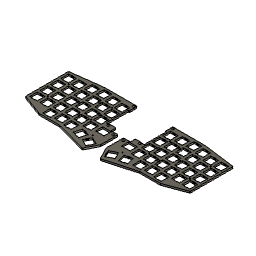
Sofle_Pico_v3.5.5_fdm_notched_plates (Autodesk Fusion 360 design; units mm, degrees)
Autodesk Fusion 360 part; units mm, degrees
sketch "Sketch1" plane through (0, 0, 0) normal (0, 0, 1) x (1, 0, 0)
  line L0 (67.7713, -100.8243) -> (105.871, -100.8243)
  line L1 (0.0502, -63.5467) -> (0.0502, -93.6294)
  arc A0 (12.757, -116.3198) -> (11.0246, -115.5539) centre (12.3611, -114.8731) cw
  arc A1 (28.6597, -14.02) -> (27.6597, -13.02) centre (28.6597, -13.02) cw
  arc A2 (27.6597, -1.075) -> (28.6597, -0.0749) centre (28.6598, -1.075) cw
  line L2 (12.7469, -62.5467) -> (12.7469, -54.5297)
  line L3 (29.4468, -54.1629) -> (29.4468, -14.02)
  line L4 (25.4468, -53.5297) -> (13.7469, -53.5297)
  line L5 (86.8212, -0.075) -> (144.1346, -7.4739)
  line L6 (105.871, -100.8243) -> (144.565, -86.5517)
  line L7 (29.4468, -54.1629) -> (26.3075, -54.1629)
  arc A3 (144.1346, -7.4739) -> (145.4707, -8.9749) centre (143.9598, -8.9748) cw
  line L8 (145.4707, -8.9749) -> (145.4707, -85.1744)
  line L9 (0.2137, -94.3371) -> (11.0246, -115.5539)
  arc A4 (12.7469, -54.5297) -> (13.7469, -53.5297) centre (13.7469, -54.5297) cw
  line L10 (1.0502, -62.5467) -> (12.7469, -62.5467)
  arc A5 (25.4468, -53.5297) -> (26.3075, -54.1629) centre (23.7986, -56.6716) cw
  line L11 (28.6597, -14.02) -> (29.4468, -14.02)
  line L12 (86.8212, -0.075) -> (28.6597, -0.075)
  arc A6 (0.2137, -94.3371) -> (0.0502, -93.6294) centre (1.5521, -93.6552) cw
  line L13 (12.757, -116.3198) -> (67.7713, -100.8243)
  line L14 (27.6597, -1.075) -> (27.6597, -13.02)
  arc A7 (145.4707, -85.1744) -> (144.565, -86.5517) centre (143.9712, -85.1747) cw
  arc A8 (0.0502, -63.5467) -> (1.0502, -62.5468) centre (1.0502, -63.5468) cw
  circle A9 centre (48.7216, -47.4698) radius 1.75
  circle A10 centre (67.7715, -28.4199) radius 1.75
  circle A11 centre (67.7715, -66.5196) radius 1.75
  circle A12 centre (86.8214, -47.4698) radius 1.75
  line L15 (26.6468, -77.0995) -> (11.0469, -77.0995)
  line L16 (11.0469, -77.0995) -> (11.0469, -64.0996)
  line L17 (11.0469, -64.0996) -> (26.6468, -64.0996)
  line L18 (26.6468, -64.0996) -> (26.6468, -77.0995)
  circle A13 centre (124.9361, -28.0099) radius 1.1
  circle A14 centre (124.9211, -66.1246) radius 1.1
  circle A15 centre (48.0866, -25.6099) radius 1.1
  circle A16 centre (48.1766, -63.5596) radius 1.1
  circle A17 centre (22.2368, -86.6295) radius 1.1
  circle A18 centre (30.6568, -3.2176) radius 2.05
  circle A19 centre (23.7868, -56.6897) radius 2.05
  circle A20 centre (4.296, -67.0996) radius 2.05
  line L19 (37.0467, -9.6) -> (41.3467, -9.6)
  line L20 (41.3467, -9.6) -> (41.3467, -8.6)
  line L21 (41.3467, -8.6) -> (37.0467, -8.6)
  line L22 (37.0467, -8.6) -> (37.0467, -9.6)
  line L23 (37.0467, -23.5999) -> (41.3467, -23.5999)
  line L24 (41.3467, -23.5999) -> (41.3467, -22.5999)
  line L25 (41.3467, -22.5999) -> (37.0467, -22.5999)
  line L26 (37.0467, -22.5999) -> (37.0467, -23.5999)
  line L27 (46.1967, -23.0999) -> (32.1968, -23.0999)
  line L28 (32.1968, -23.0999) -> (32.1968, -9.1)
  line L29 (32.1968, -9.1) -> (46.1967, -9.1)
  line L30 (46.1967, -9.1) -> (46.1967, -23.0999)
  line L31 (75.1465, -4.6001) -> (79.4464, -4.6001)
  line L32 (79.4464, -4.6001) -> (79.4464, -3.6001)
  line L33 (79.4464, -3.6001) -> (75.1465, -3.6001)
  line L34 (75.1465, -3.6001) -> (75.1465, -4.6001)
  line L35 (75.1465, -18.6) -> (79.4464, -18.6)
  line L36 (79.4464, -18.6) -> (79.4464, -17.6)
  line L37 (79.4464, -17.6) -> (75.1465, -17.6)
  line L38 (75.1465, -17.6) -> (75.1465, -18.6)
  line L39 (84.2964, -18.1) -> (70.2965, -18.1)
  line L40 (70.2965, -18.1) -> (70.2965, -4.1001)
  line L41 (70.2965, -4.1001) -> (84.2964, -4.1001)
  line L42 (84.2964, -4.1001) -> (84.2964, -18.1)
  line L43 (37.0467, -47.6998) -> (41.3467, -47.6998)
  line L44 (41.3467, -47.6998) -> (41.3467, -46.6998)
  line L45 (41.3467, -46.6998) -> (37.0467, -46.6998)
  line L46 (37.0467, -46.6998) -> (37.0467, -47.6998)
  line L47 (37.0467, -61.6997) -> (41.3467, -61.6997)
  line L48 (41.3467, -61.6997) -> (41.3467, -60.6997)
  line L49 (41.3467, -60.6997) -> (37.0467, -60.6997)
  line L50 (37.0467, -60.6997) -> (37.0467, -61.6997)
  line L51 (46.1967, -61.1997) -> (32.1968, -61.1997)
  line L52 (32.1968, -61.1997) -> (32.1968, -47.1998)
  line L53 (32.1968, -47.1998) -> (46.1967, -47.1998)
  line L54 (46.1967, -47.1998) -> (46.1967, -61.1997)
  line L55 (56.0966, -45.1998) -> (60.3966, -45.1998)
  line L56 (60.3966, -45.1998) -> (60.3966, -44.1998)
  line L57 (60.3966, -44.1998) -> (56.0966, -44.1998)
  line L58 (56.0966, -44.1998) -> (56.0966, -45.1998)
  line L59 (56.0966, -59.1997) -> (60.3966, -59.1997)
  line L60 (60.3966, -59.1997) -> (60.3966, -58.1997)
  line L61 (60.3966, -58.1997) -> (56.0966, -58.1997)
  line L62 (56.0966, -58.1997) -> (56.0966, -59.1997)
  line L63 (65.2465, -58.6997) -> (51.2466, -58.6997)
  line L64 (51.2466, -58.6997) -> (51.2466, -44.6998)
  line L65 (51.2466, -44.6998) -> (65.2465, -44.6998)
  line L66 (65.2465, -44.6998) -> (65.2465, -58.6997)
  line L67 (75.1465, -61.7496) -> (79.4464, -61.7496)
  line L68 (79.4464, -61.7496) -> (79.4464, -60.7497)
  line L69 (79.4464, -60.7497) -> (75.1465, -60.7497)
  line L70 (75.1465, -60.7497) -> (75.1465, -61.7496)
  line L71 (75.1465, -75.7495) -> (79.4464, -75.7495)
  line L72 (79.4464, -75.7495) -> (79.4464, -74.7496)
  line L73 (79.4464, -74.7496) -> (75.1465, -74.7496)
  line L74 (75.1465, -74.7496) -> (75.1465, -75.7495)
  line L75 (84.2964, -75.2496) -> (70.2965, -75.2496)
  line L76 (70.2965, -75.2496) -> (70.2965, -61.2497)
  line L77 (70.2965, -61.2497) -> (84.2964, -61.2497)
  line L78 (84.2964, -61.2497) -> (84.2964, -75.2496)
  line L79 (113.2462, -69.1496) -> (117.5461, -69.1496)
  line L80 (117.5461, -69.1496) -> (117.5461, -68.1496)
  line L81 (117.5461, -68.1496) -> (113.2462, -68.1496)
  line L82 (113.2462, -68.1496) -> (113.2462, -69.1496)
  line L83 (113.2462, -83.1495) -> (117.5461, -83.1495)
  line L84 (117.5461, -83.1495) -> (117.5461, -82.1495)
  line L85 (117.5461, -82.1495) -> (113.2462, -82.1495)
  line L86 (113.2462, -82.1495) -> (113.2462, -83.1495)
  line L87 (122.3961, -82.6495) -> (108.3962, -82.6495)
  line L88 (108.3962, -82.6495) -> (108.3962, -68.6496)
  line L89 (108.3962, -68.6496) -> (122.3961, -68.6496)
  line L90 (122.3961, -68.6496) -> (122.3961, -82.6495)
  line L91 (20.2581, -95.0736) -> (22.2101, -98.905)
  line L92 (22.2101, -98.905) -> (23.1011, -98.451)
  line L93 (23.1011, -98.451) -> (21.149, -94.6197)
  line L94 (21.149, -94.6197) -> (20.2581, -95.0736)
  line L95 (7.784, -101.4295) -> (9.7361, -105.2607)
  line L96 (9.7361, -105.2607) -> (10.6271, -104.8067)
  line L97 (10.6271, -104.8067) -> (8.675, -100.9755)
  line L98 (8.675, -100.9755) -> (7.784, -101.4295)
  line L99 (12.3835, -109.3551) -> (6.0277, -96.8811)
  line L100 (6.0277, -96.8811) -> (18.5017, -90.5253)
  line L101 (18.5017, -90.5253) -> (24.8575, -102.9993)
  line L102 (24.8575, -102.9993) -> (12.3835, -109.3551)
  line L103 (32.4877, -88.7775) -> (36.6411, -87.6646)
  line L104 (36.6411, -87.6646) -> (36.3823, -86.6986)
  line L105 (36.3823, -86.6986) -> (32.2289, -87.8116)
  line L106 (32.2289, -87.8116) -> (32.4877, -88.7775)
  line L107 (36.1111, -102.3003) -> (40.2645, -101.1874)
  line L108 (40.2645, -101.1874) -> (40.0057, -100.2215)
  line L109 (40.0057, -100.2215) -> (35.8522, -101.3344)
  line L110 (35.8522, -101.3344) -> (36.1111, -102.3003)
  line L111 (44.8199, -99.4492) -> (31.297, -103.0726)
  line L112 (31.297, -103.0726) -> (27.6735, -89.5497)
  line L113 (27.6735, -89.5497) -> (41.1964, -85.9263)
  line L114 (41.1964, -85.9263) -> (44.8199, -99.4492)
  line L115 (132.296, -31.0499) -> (136.596, -31.0499)
  line L116 (136.596, -31.0499) -> (136.596, -30.0499)
  line L117 (136.596, -30.0499) -> (132.296, -30.0499)
  line L118 (132.296, -30.0499) -> (132.296, -31.0499)
  line L119 (132.296, -45.0498) -> (136.596, -45.0498)
  line L120 (136.596, -45.0498) -> (136.596, -44.0498)
  line L121 (136.596, -44.0498) -> (132.296, -44.0498)
  line L122 (132.296, -44.0498) -> (132.296, -45.0498)
  line L123 (141.446, -44.5498) -> (127.4461, -44.5498)
  line L124 (127.4461, -44.5498) -> (127.4461, -30.5499)
  line L125 (127.4461, -30.5499) -> (141.446, -30.5499)
  line L126 (141.446, -30.5499) -> (141.446, -44.5498)
  line L127 (132.296, -50.0997) -> (136.596, -50.0997)
  line L128 (136.596, -50.0997) -> (136.596, -49.0997)
  line L129 (136.596, -49.0997) -> (132.296, -49.0997)
  line L130 (132.296, -49.0997) -> (132.296, -50.0997)
  line L131 (132.296, -64.0996) -> (136.596, -64.0996)
  line L132 (136.596, -64.0996) -> (136.596, -63.0996)
  line L133 (136.596, -63.0996) -> (132.296, -63.0996)
  line L134 (132.296, -63.0996) -> (132.296, -64.0996)
  line L135 (141.446, -63.5996) -> (127.4461, -63.5996)
  line L136 (127.4461, -63.5996) -> (127.4461, -49.5997)
  line L137 (127.4461, -49.5997) -> (141.446, -49.5997)
  line L138 (141.446, -49.5997) -> (141.446, -63.5996)
  line L139 (132.296, -69.1496) -> (136.596, -69.1496)
  line L140 (136.596, -69.1496) -> (136.596, -68.1496)
  line L141 (136.596, -68.1496) -> (132.296, -68.1496)
  line L142 (132.296, -68.1496) -> (132.296, -69.1496)
  line L143 (132.296, -83.1495) -> (136.596, -83.1495)
  line L144 (136.596, -83.1495) -> (136.596, -82.1495)
  line L145 (136.596, -82.1495) -> (132.296, -82.1495)
  line L146 (132.296, -82.1495) -> (132.296, -83.1495)
  line L147 (141.446, -82.6495) -> (127.4461, -82.6495)
  line L148 (127.4461, -82.6495) -> (127.4461, -68.6496)
  line L149 (127.4461, -68.6496) -> (141.446, -68.6496)
  line L150 (141.446, -68.6496) -> (141.446, -82.6495)
  line L151 (94.1963, -7.1) -> (98.4963, -7.1)
  line L152 (98.4963, -7.1) -> (98.4963, -6.1001)
  line L153 (98.4963, -6.1001) -> (94.1963, -6.1001)
  line L154 (94.1963, -6.1001) -> (94.1963, -7.1)
  line L155 (94.1963, -21.0999) -> (98.4963, -21.0999)
  line L156 (98.4963, -21.0999) -> (98.4963, -20.1)
  line L157 (98.4963, -20.1) -> (94.1963, -20.1)
  line L158 (94.1963, -20.1) -> (94.1963, -21.0999)
  line L159 (103.3462, -20.5999) -> (89.3463, -20.5999)
  line L160 (89.3463, -20.5999) -> (89.3463, -6.6001)
  line L161 (89.3463, -6.6001) -> (103.3462, -6.6001)
  line L162 (103.3462, -6.6001) -> (103.3462, -20.5999)
  line L163 (113.2462, -12) -> (117.5461, -12)
  line L164 (117.5461, -12) -> (117.5461, -11)
  line L165 (117.5461, -11) -> (113.2462, -11)
  line L166 (113.2462, -11) -> (113.2462, -12)
  line L167 (113.2462, -25.9999) -> (117.5461, -25.9999)
  line L168 (117.5461, -25.9999) -> (117.5461, -24.9999)
  line L169 (117.5461, -24.9999) -> (113.2462, -24.9999)
  line L170 (113.2462, -24.9999) -> (113.2462, -25.9999)
  line L171 (122.3961, -25.4999) -> (108.3962, -25.4999)
  line L172 (108.3962, -25.4999) -> (108.3962, -11.5)
  line L173 (108.3962, -11.5) -> (122.3961, -11.5)
  line L174 (122.3961, -11.5) -> (122.3961, -25.4999)
  line L175 (56.0966, -26.1499) -> (60.3966, -26.1499)
  line L176 (60.3966, -26.1499) -> (60.3966, -25.1499)
  line L177 (60.3966, -25.1499) -> (56.0966, -25.1499)
  line L178 (56.0966, -25.1499) -> (56.0966, -26.1499)
  line L179 (56.0966, -40.1498) -> (60.3966, -40.1498)
  line L180 (60.3966, -40.1498) -> (60.3966, -39.1498)
  line L181 (60.3966, -39.1498) -> (56.0966, -39.1498)
  line L182 (56.0966, -39.1498) -> (56.0966, -40.1498)
  line L183 (65.2465, -39.6498) -> (51.2466, -39.6498)
  line L184 (51.2466, -39.6498) -> (51.2466, -25.6499)
  line L185 (51.2466, -25.6499) -> (65.2465, -25.6499)
  line L186 (65.2465, -25.6499) -> (65.2465, -39.6498)
  line L187 (94.1963, -26.1499) -> (98.4963, -26.1499)
  line L188 (98.4963, -26.1499) -> (98.4963, -25.1499)
  line L189 (98.4963, -25.1499) -> (94.1963, -25.1499)
  line L190 (94.1963, -25.1499) -> (94.1963, -26.1499)
  line L191 (94.1963, -40.1498) -> (98.4963, -40.1498)
  line L192 (98.4963, -40.1498) -> (98.4963, -39.1498)
  line L193 (98.4963, -39.1498) -> (94.1963, -39.1498)
  line L194 (94.1963, -39.1498) -> (94.1963, -40.1498)
  line L195 (103.3462, -39.6498) -> (89.3463, -39.6498)
  line L196 (89.3463, -39.6498) -> (89.3463, -25.6499)
  line L197 (89.3463, -25.6499) -> (103.3462, -25.6499)
  line L198 (103.3462, -25.6499) -> (103.3462, -39.6498)
  line L199 (75.1465, -23.6499) -> (79.4464, -23.6499)
  line L200 (79.4464, -23.6499) -> (79.4464, -22.6499)
  line L201 (79.4464, -22.6499) -> (75.1465, -22.6499)
  line L202 (75.1465, -22.6499) -> (75.1465, -23.6499)
  line L203 (75.1465, -37.6498) -> (79.4464, -37.6498)
  line L204 (79.4464, -37.6498) -> (79.4464, -36.6498)
  line L205 (79.4464, -36.6498) -> (75.1465, -36.6498)
  line L206 (75.1465, -36.6498) -> (75.1465, -37.6498)
  line L207 (84.2964, -37.1498) -> (70.2965, -37.1498)
  line L208 (70.2965, -37.1498) -> (70.2965, -23.1499)
  line L209 (70.2965, -23.1499) -> (84.2964, -23.1499)
  line L210 (84.2964, -23.1499) -> (84.2964, -37.1498)
  line L211 (94.1963, -45.1998) -> (98.4963, -45.1998)
  line L212 (98.4963, -45.1998) -> (98.4963, -44.1998)
  line L213 (98.4963, -44.1998) -> (94.1963, -44.1998)
  line L214 (94.1963, -44.1998) -> (94.1963, -45.1998)
  line L215 (94.1963, -59.1997) -> (98.4963, -59.1997)
  line L216 (98.4963, -59.1997) -> (98.4963, -58.1997)
  line L217 (98.4963, -58.1997) -> (94.1963, -58.1997)
  line L218 (94.1963, -58.1997) -> (94.1963, -59.1997)
  line L219 (103.3462, -58.6997) -> (89.3463, -58.6997)
  line L220 (89.3463, -58.6997) -> (89.3463, -44.6998)
  line L221 (89.3463, -44.6998) -> (103.3462, -44.6998)
  line L222 (103.3462, -44.6998) -> (103.3462, -58.6997)
  line L223 (132.296, -12) -> (136.596, -12)
  line L224 (136.596, -12) -> (136.596, -11)
  line L225 (136.596, -11) -> (132.296, -11)
  line L226 (132.296, -11) -> (132.296, -12)
  line L227 (132.296, -25.9999) -> (136.596, -25.9999)
  line L228 (136.596, -25.9999) -> (136.596, -24.9999)
  line L229 (136.596, -24.9999) -> (132.296, -24.9999)
  line L230 (132.296, -24.9999) -> (132.296, -25.9999)
  line L231 (141.446, -25.4999) -> (127.4461, -25.4999)
  line L232 (127.4461, -25.4999) -> (127.4461, -11.5)
  line L233 (127.4461, -11.5) -> (141.446, -11.5)
  line L234 (141.446, -11.5) -> (141.446, -25.4999)
  line L235 (37.0467, -28.6499) -> (41.3467, -28.6499)
  line L236 (41.3467, -28.6499) -> (41.3467, -27.6499)
  line L237 (41.3467, -27.6499) -> (37.0467, -27.6499)
  line L238 (37.0467, -27.6499) -> (37.0467, -28.6499)
  line L239 (37.0467, -42.6498) -> (41.3467, -42.6498)
  line L240 (41.3467, -42.6498) -> (41.3467, -41.6498)
  line L241 (41.3467, -41.6498) -> (37.0467, -41.6498)
  line L242 (37.0467, -41.6498) -> (37.0467, -42.6498)
  line L243 (46.1967, -42.1498) -> (32.1968, -42.1498)
  line L244 (32.1968, -42.1498) -> (32.1968, -28.1499)
  line L245 (32.1968, -28.1499) -> (46.1967, -28.1499)
  line L246 (46.1967, -28.1499) -> (46.1967, -42.1498)
  line L247 (94.1963, -83.2995) -> (98.4963, -83.2995)
  line L248 (98.4963, -83.2995) -> (98.4963, -82.2995)
  line L249 (98.4963, -82.2995) -> (94.1963, -82.2995)
  line L250 (94.1963, -82.2995) -> (94.1963, -83.2995)
  line L251 (94.1963, -97.2994) -> (98.4963, -97.2994)
  line L252 (98.4963, -97.2994) -> (98.4963, -96.2994)
  line L253 (98.4963, -96.2994) -> (94.1963, -96.2994)
  line L254 (94.1963, -96.2994) -> (94.1963, -97.2994)
  line L255 (103.3462, -96.7994) -> (89.3463, -96.7994)
  line L256 (89.3463, -96.7994) -> (89.3463, -82.7995)
  line L257 (89.3463, -82.7995) -> (103.3462, -82.7995)
  line L258 (103.3462, -82.7995) -> (103.3462, -96.7994)
  line L259 (113.2462, -31.0499) -> (117.5461, -31.0499)
  line L260 (117.5461, -31.0499) -> (117.5461, -30.0499)
  line L261 (117.5461, -30.0499) -> (113.2462, -30.0499)
  line L262 (113.2462, -30.0499) -> (113.2462, -31.0499)
  line L263 (113.2462, -45.0498) -> (117.5461, -45.0498)
  line L264 (117.5461, -45.0498) -> (117.5461, -44.0498)
  line L265 (117.5461, -44.0498) -> (113.2462, -44.0498)
  line L266 (113.2462, -44.0498) -> (113.2462, -45.0498)
  line L267 (122.3961, -44.5498) -> (108.3962, -44.5498)
  line L268 (108.3962, -44.5498) -> (108.3962, -30.5499)
  line L269 (108.3962, -30.5499) -> (122.3961, -30.5499)
  line L270 (122.3961, -30.5499) -> (122.3961, -44.5498)
  line L271 (94.1963, -64.2496) -> (98.4963, -64.2496)
  line L272 (98.4963, -64.2496) -> (98.4963, -63.2496)
  line L273 (98.4963, -63.2496) -> (94.1963, -63.2496)
  line L274 (94.1963, -63.2496) -> (94.1963, -64.2496)
  line L275 (94.1963, -78.2495) -> (98.4963, -78.2495)
  line L276 (98.4963, -78.2495) -> (98.4963, -77.2495)
  line L277 (98.4963, -77.2495) -> (94.1963, -77.2495)
  line L278 (94.1963, -77.2495) -> (94.1963, -78.2495)
  line L279 (103.3462, -77.7495) -> (89.3463, -77.7495)
  line L280 (89.3463, -77.7495) -> (89.3463, -63.7496)
  line L281 (89.3463, -63.7496) -> (103.3462, -63.7496)
  line L282 (103.3462, -63.7496) -> (103.3462, -77.7495)
  line L283 (113.2462, -50.0997) -> (117.5461, -50.0997)
  line L284 (117.5461, -50.0997) -> (117.5461, -49.0997)
  line L285 (117.5461, -49.0997) -> (113.2462, -49.0997)
  line L286 (113.2462, -49.0997) -> (113.2462, -50.0997)
  line L287 (113.2462, -64.0996) -> (117.5461, -64.0996)
  line L288 (117.5461, -64.0996) -> (117.5461, -63.0996)
  line L289 (117.5461, -63.0996) -> (113.2462, -63.0996)
  line L290 (113.2462, -63.0996) -> (113.2462, -64.0996)
  line L291 (122.3961, -63.5996) -> (108.3962, -63.5996)
  line L292 (108.3962, -63.5996) -> (108.3962, -49.5997)
  line L293 (108.3962, -49.5997) -> (122.3961, -49.5997)
  line L294 (122.3961, -49.5997) -> (122.3961, -63.5996)
  line L295 (75.1465, -80.7995) -> (79.4464, -80.7995)
  line L296 (79.4464, -80.7995) -> (79.4464, -79.7995)
  line L297 (79.4464, -79.7995) -> (75.1465, -79.7995)
  line L298 (75.1465, -79.7995) -> (75.1465, -80.7995)
  line L299 (75.1465, -94.7994) -> (79.4464, -94.7994)
  line L300 (79.4464, -94.7994) -> (79.4464, -93.7994)
  line L301 (79.4464, -93.7994) -> (75.1465, -93.7994)
  line L302 (75.1465, -93.7994) -> (75.1465, -94.7994)
  line L303 (84.2964, -94.2994) -> (70.2965, -94.2994)
  line L304 (70.2965, -94.2994) -> (70.2965, -80.2995)
  line L305 (70.2965, -80.2995) -> (84.2964, -80.2995)
  line L306 (84.2964, -80.2995) -> (84.2964, -94.2994)
  line L307 (75.1465, -42.6998) -> (79.4464, -42.6998)
  line L308 (79.4464, -42.6998) -> (79.4464, -41.6998)
  line L309 (79.4464, -41.6998) -> (75.1465, -41.6998)
  line L310 (75.1465, -41.6998) -> (75.1465, -42.6998)
  line L311 (75.1465, -56.6997) -> (79.4464, -56.6997)
  line L312 (79.4464, -56.6997) -> (79.4464, -55.6997)
  line L313 (79.4464, -55.6997) -> (75.1465, -55.6997)
  line L314 (75.1465, -55.6997) -> (75.1465, -56.6997)
  line L315 (84.2964, -56.1997) -> (70.2965, -56.1997)
  line L316 (70.2965, -56.1997) -> (70.2965, -42.1998)
  line L317 (70.2965, -42.1998) -> (84.2964, -42.1998)
  line L318 (84.2964, -42.1998) -> (84.2964, -56.1997)
  line L319 (56.0966, -7.1) -> (60.3966, -7.1)
  line L320 (60.3966, -7.1) -> (60.3966, -6.1001)
  line L321 (60.3966, -6.1001) -> (56.0966, -6.1001)
  line L322 (56.0966, -6.1001) -> (56.0966, -7.1)
  line L323 (56.0966, -21.0999) -> (60.3966, -21.0999)
  line L324 (60.3966, -21.0999) -> (60.3966, -20.1)
  line L325 (60.3966, -20.1) -> (56.0966, -20.1)
  line L326 (56.0966, -20.1) -> (56.0966, -21.0999)
  line L327 (65.2465, -20.5999) -> (51.2466, -20.5999)
  line L328 (51.2466, -20.5999) -> (51.2466, -6.6001)
  line L329 (51.2466, -6.6001) -> (65.2465, -6.6001)
  line L330 (65.2465, -6.6001) -> (65.2465, -20.5999)
  line L331 (56.0966, -64.2496) -> (60.3966, -64.2496)
  line L332 (60.3966, -64.2496) -> (60.3966, -63.2496)
  line L333 (60.3966, -63.2496) -> (56.0966, -63.2496)
  line L334 (56.0966, -63.2496) -> (56.0966, -64.2496)
  line L335 (56.0966, -78.2495) -> (60.3966, -78.2495)
  line L336 (60.3966, -78.2495) -> (60.3966, -77.2495)
  line L337 (60.3966, -77.2495) -> (56.0966, -77.2495)
  line L338 (56.0966, -77.2495) -> (56.0966, -78.2495)
  line L339 (65.2465, -77.7495) -> (51.2466, -77.7495)
  line L340 (51.2466, -77.7495) -> (51.2466, -63.7496)
  line L341 (51.2466, -63.7496) -> (65.2465, -63.7496)
  line L342 (65.2465, -63.7496) -> (65.2465, -77.7495)
  line L343 (56.0966, -83.2995) -> (60.3966, -83.2995)
  line L344 (60.3966, -83.2995) -> (60.3966, -82.2995)
  line L345 (60.3966, -82.2995) -> (56.0966, -82.2995)
  line L346 (56.0966, -82.2995) -> (56.0966, -83.2995)
  line L347 (56.0966, -97.2994) -> (60.3966, -97.2994)
  line L348 (60.3966, -97.2994) -> (60.3966, -96.2994)
  line L349 (60.3966, -96.2994) -> (56.0966, -96.2994)
  line L350 (56.0966, -96.2994) -> (56.0966, -97.2994)
  line L351 (65.2465, -96.7994) -> (51.2466, -96.7994)
  line L352 (51.2466, -96.7994) -> (51.2466, -82.7995)
  line L353 (51.2466, -82.7995) -> (65.2465, -82.7995)
  line L354 (65.2465, -82.7995) -> (65.2465, -96.7994)
  line L355 (37.0467, -66.7496) -> (41.3467, -66.7496)
  line L356 (41.3467, -66.7496) -> (41.3467, -65.7496)
  line L357 (41.3467, -65.7496) -> (37.0467, -65.7496)
  line L358 (37.0467, -65.7496) -> (37.0467, -66.7496)
  line L359 (37.0467, -80.7495) -> (41.3467, -80.7495)
  line L360 (41.3467, -80.7495) -> (41.3467, -79.7495)
  line L361 (41.3467, -79.7495) -> (37.0467, -79.7495)
  line L362 (37.0467, -79.7495) -> (37.0467, -80.7495)
  line L363 (46.1967, -80.2495) -> (32.1968, -80.2495)
  line L364 (32.1968, -80.2495) -> (32.1968, -66.2496)
  line L365 (32.1968, -66.2496) -> (46.1967, -66.2496)
  line L366 (46.1967, -66.2496) -> (46.1967, -80.2495)
  line L367 (-8.0971, 10.0635) -> (157.3145, 10.0635)
  line L368 (157.3145, 10.0635) -> (157.3145, -126.4299)
  line L369 (157.3145, -126.4299) -> (-8.0971, -126.4299)
  line L370 (-8.0971, -126.4299) -> (-8.0971, 10.0635)
  line L371 (67.7713, -100.8243) -> (67.7713, -126.4299)
  line L372 (105.871, -100.8243) -> (105.871, -126.4299)
  line L373 (145.4707, -85.1744) -> (157.3145, -85.1744)
  line L374 (144.1346, -7.4739) -> (144.1346, 10.0635)
  line L375 (28.6597, -0.0749) -> (28.6597, 10.0635)
  line L376 (12.7469, -54.5297) -> (-8.0971, -54.5297)
  line L377 (0.0502, -93.6294) -> (-8.0971, -93.6294)
  line L378 (0.0502, -63.5467) -> (-8.0971, -63.5467)
  line L379 (1.0502, -62.5467) -> (1.0502, -54.5297)
  circle A21 centre (1.0502, -63.5468) radius 1.0001
  line L380 (86.8212, -0.075) -> (86.8212, 10.0635)
  circle A22 centre (28.6598, -1.075) radius 1
  line L381 (28.6597, -0.0749) -> (86.8212, -0.075)
  point P0 (50.4716, -47.4698)
  point P1 (69.5215, -28.4199)
  point P2 (69.5215, -66.5196)
  point P3 (88.5714, -47.4698)
  point P4 (126.0361, -28.0099)
  point P5 (126.0211, -66.1246)
  point P6 (49.1866, -25.6099)
  point P7 (49.2766, -63.5596)
  point P8 (23.3368, -86.6295)
  point P9 (32.7068, -3.2176)
  point P10 (25.8368, -56.6897)
  point P11 (6.346, -67.0996)
  constraint horizontal L367
  constraint vertical L368
  constraint horizontal L369
  constraint vertical L370
  constraint coincident L369 L371.end
  constraint perpendicular L369 L371
  constraint coincident L369 L372.end
  constraint perpendicular L369 L372
  constraint coincident L368 L373.end
  constraint perpendicular L368 L373
  constraint coincident L367 L374.end
  constraint perpendicular L367 L374
  constraint coincident L367 L375.end
  constraint perpendicular L367 L375
  constraint coincident L370 L376.end
  constraint perpendicular L370 L376
  constraint coincident L370 L377.end
  constraint perpendicular L370 L377
  constraint coincident L370 L378.end
  constraint perpendicular L370 L378
  constraint coincident L376 L379.end
  constraint perpendicular L376 L379
  constraint concentric A8 A21
  constraint coincident L10.start A21
  constraint coincident L367 L380.end
  constraint perpendicular L367 L380
  constraint concentric A2 A22
  constraint coincident L12.end A22
extrude "Extrude1" add sketch "Sketch1" against normal blind 1.5 contours L0 L1 A0 A1 L2 L3 L4 L5 L6 L7 A3 L8 L9 A4 L10 A5 L11 L12 A6 L13 L14 A7 A18 A21 A22 L381 | A8 A21 | A2 A18 A22 | L20 L21 L22 L29 | L23 L24 L26 L27 | L32 L33 L34 L41 | L35 L36 L38 L39 | L44 L45 L46 L53 | L47 L48 L50 L51 | L56 L57 L58 L65 | L59 L60 L62 L63 | L68 L69 L70 L77 | L71 L72 L74 L75 | L80 L81 L82 L89 | L83 L84 L86 L87 | L92 L93 L94 L101 | L95 L96 L98 L99 | L104 L105 L106 L113 | L107 L108 L110 L111 | L116 L117 L118 L125 | L119 L120 L122 L123 | L128 L129 L130 L137 | L131 L132 L134 L135 | L140 L141 L142 L149 | L143 L144 L146 L147 | L152 L153 L154 L161 | L155 L156 L158 L159 | L164 L165 L166 L173 | L167 L168 L170 L171 | L176 L177 L178 L185 | L179 L180 L182 L183 | L188 L189 L190 L197 | L191 L192 L194 L195 | L200 L201 L202 L209 | L203 L204 L206 L207 | L212 L213 L214 L221 | L215 L216 L218 L219 | L224 L225 L226 L233 | L227 L228 L230 L231 | L236 L237 L238 L245 | L239 L240 L242 L243 | L248 L249 L250 L257 | L251 L252 L254 L255 | L260 L261 L262 L269 | L263 L264 L266 L267 | L272 L273 L274 L281 | L275 L276 L278 L279 | L284 L285 L286 L293 | L287 L288 L290 L291 | L296 L297 L298 L305 | L299 L300 L302 L303 | L308 L309 L310 L317 | L311 L312 L314 L315 | L320 L321 L322 L329 | L323 L324 L326 L327 | L332 L333 L334 L341 | L335 L336 L338 L339 | L344 L345 L346 L353 | L347 L348 L350 L351 | L356 L357 L358 L365 | L359 L360 L362 L363 makes body 1
extrude "Extrude2" add sketch "Sketch1" along normal blind 1.5 contours L0 L1 A0 A1 L2 L3 L4 L5 L6 L7 A3 L8 L9 A4 L10 A5 L11 L12 A6 L13 L14 A7 A18 A21 A22 L381 | A8 A21 | A2 A18 A22 bodies 1
ref_plane "WorkPlane1" through (-5, 0, 0) normal (1, 0, 0) x (0, 1, 0)
mirror "Mirror1" about plane through (-5, 0, 0) normal (1, 0, 0) of bodies 1 makes body 2
equation "retention_nub_depth = 1.5 mm"
equation "plate_thickness = 3 mm"
equation "d3 = -retention_nub_depth"
equation "d5 = plate_thickness - retention_nub_depth"
named bodies: "LH_thick_keyplate_sofle_pico_v3.5.5", "RH_thick_keyplate_sofle_pico_v3.5.5"
